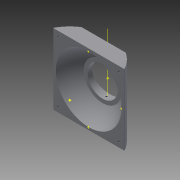
# Autodesk Inventor part: Custom Mirror Design Part 2
Saved by Autodesk Inventor 2015 (Build 190159000, 159)
## iProperties
Created: 2014-09-08
Part Number: Custom Mirror Design Part 2
Material: Generic
Document SubType Name: Modeling
Designer: I Rabey
Density: 1 g/cm^3
Appearance: Default
Author: I Rabey
Autodesk Inventor part; units mm, degrees
ref_plane "XZ Plane" through (0, 0, 0) normal (0, 1, 0) x (-1, 0, 0)
sketch "Sketch1" plane through (0, 0, 0) normal (0, 0, 1) x (1, 0, 0)
  line L0 (65, -65) -> (-65, -65)
  line L1 (-65, -65) -> (-65, 65)
  line L2 (-65, 65) -> (65, 65)
  line L3 (65, 65) -> (65, -65)
  line L4 (65, -65) -> (-65, 65) construction
  line L5 (-65, -65) -> (65, 65) construction
  point P0 (0, 0)
  dimension "d0" = 130
  dimension "d1" = 130
  constraints: 12 end point, 2 midpoint, 2 parallel, 1 horizontal, 1 perpendicular
  measures "d0" distance of L1.end L2.end
  measures "d1" distance of L0.end L1.end
extrude "Extrusion1" add sketch "Sketch1" against normal blind 100
sketch "Sketch2" plane through (0, 0, 0) normal (0, 0, 1) x (1, 0, 0)
  arc A0 (0, 75) -> (0, -75) centre (0, 0) ccw
  line L0 (0, 0) -> (0, 75) construction
  line L1 (0, 0) -> (75, 0) construction
  line L2 (0, 0) -> (0, -75) construction
  line L3 (0, 75) -> (0, -75)
  dimension "d4" = 75
  dimension "d5" = 90
  dimension "d6" = 180
  constraints: 8 end point, 2 point on circle, 1 centre point, 1 coincident, 1 horizontal, 1 perpendicular
  measures "d4" radius of A0
  measures "d5" angle of L1 L0
  measures "d6" angle of L2 L0
revolve "Revolution1" cut sketch "Sketch2" angle 180 about axis through (0, 75, 0) along (0, -1, 0)
ref_plane "Work Plane1" through (0, 65, -37.4166) normal (0, 0, 1) x (1, 0, 0)
sketch "Sketch3" plane through (0, 65, -37.4166) normal (0, 0, 1) x (1, 0, 0)
  line L0 (-65, -130) -> (65, -130)
  line L1 (65, -130) -> (65, 0)
  line L2 (65, 0) -> (-65, 0)
  line L3 (-65, 0) -> (-65, -130)
  line L4 (-65, -130) -> (65, 0) construction
  line L5 (65, -130) -> (-65, 0) construction
  point P0 (0, -65)
  dimension "d8" = 130
  dimension "d9" = 130
  constraints: 12 end point, 2 midpoint, 2 parallel, 1 horizontal, 1 perpendicular
  measures "d8" distance of L2.end L1.end
  measures "d9" distance of L1.end L0.end
extrude "Extrusion2" cut sketch "Sketch3" along normal blind 100
sketch "Sketch4" plane through (0, 65, -37.4166) normal (0, 0, 1) x (1, 0, 0)
  line L0 (-65, -130) -> (65, -130)
  line L1 (65, -130) -> (65, 0)
  line L2 (65, 0) -> (-65, 0)
  line L3 (-65, 0) -> (-65, -130)
  line L4 (-65, -130) -> (65, 0) construction
  line L5 (65, -130) -> (-65, 0) construction
  line L6 (-70, -135) -> (70, -135)
  line L7 (70, -135) -> (70, 5)
  line L8 (70, 5) -> (-70, 5)
  line L9 (-70, 5) -> (-70, -135)
  arc A0 (65, -65) -> (0, 0) centre (0, -65) ccw projected
  line L10 (-70, -135) -> (70, 5) construction
  line L11 (70, -135) -> (-70, 5) construction
  dimension "d12" = 130
  dimension "d13" = 130
  dimension "d14" = 140
  dimension "d15" = 140
  constraints: 24 end point, 4 midpoint, 4 parallel, 2 horizontal, 2 perpendicular
  measures "d12" distance of L2.end L1.end
  measures "d13" distance of L1.end L0.end
  measures "d14" distance of L8.end L7.end
  measures "d15" distance of L7.end L6.end
extrude "Extrusion3" add sketch "Sketch4" against normal blind 50
sketch "Sketch5" plane through (-65, 65, -100) normal (0, 1, 0) x (1, 0, 0)
  line L0 (0, 0) -> (130, 0)
  line L1 (130, 0) -> (130, -12.5834)
  line L2 (130, -12.5834) -> (0, -12.5834)
  line L3 (0, -12.5834) -> (0, 0)
  point P0 (65, -100)
  constraints: 8 end point, 2 parallel, 1 horizontal, 1 perpendicular
extrude "Extrusion4" cut sketch "Sketch5" against normal blind 130
ref_plane "Work Plane2" through (0, 0, -75) normal (0, 0, 1) x (1, 0, 0)
sketch "Sketch6" plane through (0, 0, -75) normal (0, 0, 1) x (1, 0, 0)
  circle A0 centre (0, 0) radius 30
  dimension "d20" = 60
  constraints: 1 centre point, 1 coincident
  measures "d20" diameter of A0
extrude "Extrusion5" cut sketch "Sketch6" against normal blind 30 and the other way blind 30
sketch "Sketch7" plane through (0, 0, 0) normal (0, 1, 0) x (-1, 0, 0)
  circle A0 centre (0, 0) radius 80
  circle A1 centre (0, 0) radius 150
  dimension "d25" = 160
  dimension "d26" = 300
  constraints: 2 centre point, 2 coincident
  measures "d25" diameter of A0
  measures "d26" diameter of A1
extrude "Extrusion6" cut sketch "Sketch7" against normal blind 100 and the other way blind 100
sketch "Sketch8" plane through (0, 0, 0) normal (1, 0, 0) x (0, 1, 0)
  point P0 (0, 0)
ref_plane "Work Plane3" through (65, 0, -37.4166) normal (1, 0, 0) x (0, 1, 0)
sketch "Sketch10" plane through (0, 65, -37.4166) normal (0, 0, 1) x (1, 0, 0)
  circle A0 centre (-60.1041, -4.8959) radius 2
  point P0 (0, -65)
  dimension "d36" = 4
  dimension "d37" = 85
  dimension "d38" = 60.1041
  constraints: 1 centre point
  measures "d36" diameter of A0
  measures "d37" distance of point (0, -65) A0.centre
  measures "d38" horizontal distance of point (0, -65) A0.centre
sketch "Sketch11" plane through (0, 65, -37.4166) normal (0, 0, 1) x (1, 0, 0)
  circle A0 centre (60.1041, -4.8959) radius 2
  point P0 (0, -65)
  dimension "d39" = 4
  dimension "d40" = 85
  dimension "d41" = 60.1041
  constraints: 1 centre point
  measures "d39" diameter of A0
  measures "d40" distance of A0.centre point (0, -65)
  measures "d41" horizontal distance of A0.centre point (0, -65)
sketch "Sketch12" plane through (0, 65, -37.4166) normal (0, 0, 1) x (1, 0, 0)
  circle A0 centre (-60.1041, -125.1041) radius 2
  point P0 (0, -65)
  dimension "d42" = 4
  dimension "d43" = 85
  dimension "d44" = 60.1041
  constraints: 1 centre point
  measures "d42" diameter of A0
  measures "d43" distance of point (0, -65) A0.centre
  measures "d44" horizontal distance of A0.centre point (0, -65)
sketch "Sketch13" plane through (0, 65, -37.4166) normal (0, 0, 1) x (1, 0, 0)
  circle A0 centre (60.1041, -125.1041) radius 2
  point P0 (0, -65)
  dimension "d45" = 4
  dimension "d46" = 85
  dimension "d47" = 60.1041
  constraints: 1 centre point
  measures "d45" diameter of A0
  measures "d46" distance of point (0, -65) A0.centre
  measures "d47" horizontal distance of A0.centre point (0, -65)
hole "Hole1" at (-60.1041, 60.1041, -37.4166) direction (0, 0, -1) diameter 4 depth 5 tip angle 118
hole "Hole2" at (60.1041, 60.1041, -37.4166) direction (0, 0, -1) diameter 4 depth 5 tip angle 118
hole "Hole3" at (-60.1041, -60.1041, -37.4166) direction (0, 0, -1) diameter 4 depth 5 tip angle 118
hole "Hole4" at (60.1041, -60.1041, -37.4166) direction (0, 0, -1) diameter 4 depth 5 tip angle 118
thread "Thread1" size "M4x0.7" class "6H" standard "ANSI Metric M Profile" full length
thread "Thread2" size "M4x0.7" class "6H" standard "ANSI Metric M Profile" full length
thread "Thread3" size "M4x0.7" class "6H" standard "ANSI Metric M Profile" full length
thread "Thread4" size "M4x0.7" class "6H" standard "ANSI Metric M Profile" full length
ref_plane "Work Plane4" through (-70, 30, -37.4166) normal (0, 1, 0) x (1, 0, 0)
ref_plane "Work Plane5" through (0, 0, -65) normal (0, 0, 1) x (1, 0, 0)
sketch "Sketch15" plane through (0, 0, -65) normal (0, 0, 1) x (1, 0, 0)
  circle A0 centre (0, 0) radius 37.4378
  circle A1 centre (0, 0) radius 30
  dimension "d93" = 60
  constraints: 2 centre point, 2 coincident
  measures "d93" diameter of A1
extrude "Extrusion9" add sketch "Sketch15" against normal blind 40
sketch "Sketch16" plane through (0, 0, 0) normal (0, 1, 0) x (-1, 0, 0)
  circle A0 centre (0, 0) radius 80
  circle A1 centre (0, 0) radius 150
  dimension "d96" = 160
  dimension "d97" = 300
  constraints: 2 centre point, 2 coincident
  measures "d96" diameter of A0
  measures "d97" diameter of A1
extrude "Extrusion10" cut sketch "Sketch16" along normal blind 100 and the other way blind 100
sketch "Sketch17" plane through (-70, 30, -37.4166) normal (0, 1, 0) x (1, 0, 0)
  circle A0 centre (69.7648, 35.0834) radius 1.5
  line L0 (100, 27.5834) -> (40, 27.5834) projected
  point P0 (70, -37.4166)
  dimension "d102" = 3
  dimension "d103" = 7.5
  constraints: 1 centre point
  measures "d102" diameter of A0
  measures "d103" distance from line of A0.centre L0
extrude "Extrusion11" cut sketch "Sketch17" along normal blind 100 and the other way blind 2
thread "Thread7" size "M3x0.5" class "6H" standard "ANSI Metric M Profile" full length
sketch "Sketch19" plane through (-70, 70, -37.4166) normal (0, 1, 0) x (1, 0, 0)
  line L0 (20, 55.5834) -> (120, 55.5834)
  line L1 (120, 55.5834) -> (120, 29.5834)
  line L2 (120, 29.5834) -> (20, 29.5834)
  line L3 (20, 29.5834) -> (20, 55.5834)
  arc A0 (140, 1.3133) -> (0, 1.3133) centre (70, -37.4166) ccw projected
  line L4 (20, 55.5834) -> (120, 29.5834) construction
  line L5 (120, 55.5834) -> (20, 29.5834) construction
  point P0 (70, 42.5834)
  dimension "d114" = 100
  dimension "d115" = 26
  constraints: 12 end point, 2 midpoint, 2 parallel, 1 horizontal, 1 perpendicular, 1 point on circle
  measures "d114" distance of L1.end L2.end
  measures "d115" distance of L0.end L1.end
extrude "Extrusion12" cut sketch "Sketch19" against normal blind 30
sketch "Sketch20" plane through (-70, -70, -37.4166) normal (0, -1, 0) x (1, 0, 0)
  line L0 (20, -55.5834) -> (120, -55.5834)
  line L1 (120, -55.5834) -> (120, -29.5834)
  line L2 (120, -29.5834) -> (20, -29.5834)
  line L3 (20, -29.5834) -> (20, -55.5834)
  arc A0 (26.285, -29.5834) -> (113.715, -29.5834) centre (70, 37.4166) ccw projected
  line L4 (20, -55.5834) -> (120, -29.5834) construction
  line L5 (120, -55.5834) -> (20, -29.5834) construction
  point P0 (70, -42.5834)
  dimension "d118" = 100
  dimension "d119" = 26
  constraints: 12 end point, 2 midpoint, 2 parallel, 1 horizontal, 1 perpendicular, 1 point on circle
  measures "d118" distance of L2.end L1.end
  measures "d119" distance of L1.end L0.end
extrude "Extrusion13" cut sketch "Sketch20" against normal blind 30
ref_plane "Work Plane6" through (-70, -30, -37.4166) normal (0, 1, 0) x (1, 0, 0)
sketch "Sketch21" plane through (-70, -30, -37.4166) normal (0, 1, 0) x (1, 0, 0)
  circle A0 centre (70, 35.0834) radius 1.5
  line L0 (100, 27.5834) -> (40, 27.5834) projected
  point P0 (70, -37.4166)
  dimension "d123" = 3
  dimension "d130" = 7.5
  constraints: 1 centre point
  measures "d123" diameter of A0
  measures "d130" distance from line of A0.centre L0
extrude "Extrusion14" cut sketch "Sketch21" along normal blind 5 and the other way blind 100
thread "Thread8" size "M3x0.5" class "6H" standard "ANSI Metric M Profile" full length
equation "\"d0\" = d1"
equation "\"d9\" = d8"
body "Solid1"
